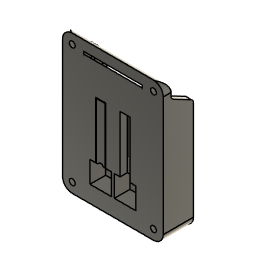
makita_10.8v_v38 v10 (Autodesk Fusion 360 design; units mm, degrees)
Autodesk Fusion 360 part; units mm, degrees
note: some values were not read from the file. Chosen so that the rebuilt part matches the saved one: a side; which face or edge a step refers to. Set by a fixed rule: which sketch regions a step uses.
(part 1 of 2)
sketch "スケッチ1" plane through (0, 0, 0) normal (0, 1, 0) x (1, 0, 0)
  line L0 (0, 0) -> (-15, 0)
  line L1 (-15, 0) -> (-15, 24)
  line L2 (-15, 24) -> (15, 24)
  line L3 (15, 24) -> (15, 0)
  line L4 (15, 0) -> (0, 0)
  line L5 (0, 0) -> (0, 36) construction
  line L6 (0, 0) -> (0, -57) construction
  line L7 (0.5, -4.15) -> (-0.5, -4.15)
  line L8 (-0.5, -4.15) -> (-0.5, -10.3)
  line L9 (-0.5, -10.3) -> (0.5, -10.3)
  line L10 (0.5, -10.3) -> (0.5, -4.15)
  line L11 (0.5, -4.15) -> (-0.5, -10.3) construction
  line L12 (-0.5, -4.15) -> (0.5, -10.3) construction
  line L13 (-6.75, 0) -> (-5.75, 0)
  line L14 (-5.75, 0) -> (-5.75, -19.4)
  line L15 (-5.75, -19.4) -> (-6.75, -19.4)
  line L16 (-6.75, -19.4) -> (-6.75, 0)
  line L17 (-6.75, -9.84) -> (-5.75, -9.84)
  line L18 (6.75, -19.4) -> (6.75, 0)
  line L19 (5.75, 0) -> (5.75, -19.4)
  line L20 (5.75, -19.4) -> (6.75, -19.4)
  line L21 (6.75, 0) -> (5.75, 0)
  line L22 (22.83, 24) -> (-22.83, 24)
  line L23 (-22.83, 24) -> (-22.83, -44.15)
  line L24 (-22.83, -44.15) -> (22.83, -44.15)
  line L25 (22.83, -44.15) -> (22.83, 24)
  line L26 (25.83, -44.15) -> (25.83, 27)
  line L27 (25.83, 27) -> (-25.83, 27)
  line L28 (-25.83, 27) -> (-25.83, -44.15)
  line L29 (-22.83, -44.15) -> (-25.83, -44.15)
  line L30 (22.83, -44.15) -> (25.83, -44.15)
  line L31 (-22.83, 1) -> (-18.63, 1)
  line L32 (-18.63, 1) -> (-18.63, -25)
  line L33 (-18.63, -25) -> (-22.83, -25)
  line L34 (-18.63, 1) -> (-18.63, 24)
  line L35 (18.63, 1) -> (18.63, 24)
  line L36 (22.83, 1) -> (18.63, 1)
  line L37 (18.63, 1) -> (18.63, -25)
  line L38 (18.63, -25) -> (22.83, -25)
  line L39 (6.75, -9.84) -> (5.75, -9.84)
  point P0 (0, -7.225)
  point P1 (0, 1.51)
  dimension "d1" = 30
  dimension "d2" = 24
  dimension "d3" = 1
  dimension "d4" = 1
  dimension "d5" = 6.15
  dimension "d6" = 19.4
  dimension "d7" = 4.15
  dimension "d8" = 5.25
  dimension "d9" = 9.56
  dimension "d10" = 45.66
  dimension "d11" = 44.15
  dimension "d12" = 3
  dimension "d13" = 1
  dimension "d14" = 26
  dimension "d15" = 7.2
  constraint coincident L0.start L4.end
  constraint horizontal L0
  constraint perpendicular L0 L1
  constraint perpendicular L1 L2
  constraint perpendicular L2 L3
  constraint perpendicular L1 L4
  constraint perpendicular L2 L5
  constraint perpendicular L0 L6
  constraint perpendicular L7 L8
  constraint parallel L7 L9
  constraint parallel L8 L10
  constraint horizontal L7
  constraint coincident L11 P0
  constraint coincident L12 P0
  constraint coincident L6 P0
  constraint horizontal L13
  constraint vertical L14
  constraint horizontal L15
  constraint vertical L16
  constraint coincident L0 L13.start
  constraint coincident L16 L17.start
  constraint coincident L14 L17.end
  constraint perpendicular L16 L17
  constraint symmetric L6 L13.start L18.end
  constraint symmetric L6 L13.end L19.start
  constraint symmetric L6 L14.end L19.end
  constraint symmetric L6 L15.end L18.start
  constraint perpendicular L22 L23
  constraint parallel L22 L24
  constraint parallel L23 L25
  constraint horizontal L22
  constraint coincident L6 P1
  constraint symmetric L6 L23 L25
  constraint collinear L2 L22
  constraint coincident L23 L31.start
  constraint perpendicular L23 L31
  constraint perpendicular L31 L32
  constraint coincident L23 L33.end
  constraint perpendicular L23 L33
  constraint coincident L22 L34.end
  constraint perpendicular L22 L34
  constraint symmetric L5 L31.start L36.start
  constraint symmetric L5 L31.end L35.start
  constraint symmetric L5 L32.end L37.end
  constraint symmetric L5 L33.end L38.end
  constraint symmetric L5 L34.end L35.end
  constraint vertical L6
  constraint symmetric L6 L17.start L39.start
  constraint symmetric L6 L17.end L39.end
  measures "d1" distance of L1 L3
  measures "d2" vertical distance of L0.end L1.end
  measures "d3" horizontal distance of L8.end L9.end
  measures "d4" horizontal distance of L14.end L15.end
  measures "d5" vertical distance of L7.end L8.end
  measures "d6" vertical distance of L13.start L15.end
  measures "d7" distance of L4 L7
  measures "d8" distance of L8 L14
  measures "d9" distance of L15 L17
  measures "d10" horizontal distance of L23.end L24.end
  measures "d11" distance of L4 L24
  measures "d13" distance of L0 L31
  measures "d14" vertical distance of L31.end L32.end
  measures "d15" distance of L28 L32
extrude "押し出し1" add sketch "スケッチ1" along normal blind 8 contours L0 L1 L2 L3 L4 L13 L21 L22 makes body 1
extrude "押し出し2" add sketch "スケッチ1" along normal blind 11.5 contours L2 L22 L23 L25 L26 L27 L28 L29 L30 | L23 L31 L32 L33 | L25 L36 L37 L38 bodies 1
extrude "押し出し3" cut sketch "スケッチ1" along normal blind 6.5 contours L22 L23 L31 L34 | L22 L25 L35 L36 | L23 L31 L32 L33 | L25 L36 L37 L38 bodies 1
extrude "押し出し4" add sketch "スケッチ1" against normal blind 4 contours L0 L1 L3 L4 L14 L15 L16 L18 L19 L20 L22 L23 L24 L25 L32 L33 L34 L35 L37 L38 | L0 L1 L2 L3 L4 L13 L21 L22 | L0 L13 L14 L16 L17 | L4 L18 L19 L21 L39 | L14 L15 L16 L17 | L18 L19 L20 L39 | L2 L22 L23 L25 L26 L27 L28 L29 L30 | L22 L23 L31 L34 | L22 L25 L35 L36 | L23 L31 L32 L33 | L25 L36 L37 L38 | L7 L8 L9 L10 bodies 1
extrude "押し出し5" cut sketch "スケッチ1" against normal up to surface (4 mm away) contours L14 L15 L16 L17 | L18 L19 L20 L39 bodies 1
sketch "スケッチ2" plane through (0, 0, 0) normal (0, 1, 0) x (-1, 0, 0)
  line L0 (-5.75, 19.4) -> (-5.75, 9.84)
  line L1 (-5.75, 9.84) -> (-6.75, 9.84)
  line L2 (-6.75, 9.84) -> (-6.75, 19.4)
  line L3 (-6.75, 19.4) -> (-5.75, 19.4)
  line L4 (5.75, 19.4) -> (6.75, 19.4)
  line L5 (6.75, 19.4) -> (6.75, 9.84)
  line L6 (6.75, 9.84) -> (5.75, 9.84)
  line L7 (5.75, 9.84) -> (5.75, 19.4)
  line L8 (-22.83, 44.15) -> (-22.83, -24)
  line L9 (-22.83, -24) -> (-15, -24)
  line L10 (-15, -24) -> (-15, 0)
  line L11 (-15, 0) -> (0, 0)
  line L12 (0, 0) -> (5.75, 0)
  line L13 (5.75, 0) -> (6.75, 0)
  line L14 (6.75, 0) -> (15, 0)
  line L15 (15, 0) -> (15, -24)
  line L16 (15, -24) -> (22.83, -24)
  line L17 (22.83, -24) -> (22.83, 44.15)
  line L18 (22.83, 44.15) -> (-22.83, 44.15)
  line L19 (6.75, 19.4) -> (6.75, 9.84)
  line L20 (5.75, 9.84) -> (5.75, 19.4)
  line L21 (-5.75, 19.4) -> (-5.75, 9.84)
  line L22 (-6.75, 9.84) -> (-6.75, 19.4)
  line L23 (8.175, 21.4) -> (4.325, 21.4)
  line L24 (4.325, 21.4) -> (4.325, 0)
  line L25 (4.325, 0) -> (8.175, 0)
  line L26 (8.175, 0) -> (8.175, 21.4)
  line L27 (6.25, 9.84) -> (6.25, 19.4) construction
  line L28 (0, 0) -> (0, 25.4511) construction
  line L29 (-8.175, 0) -> (-8.175, 21.4)
  line L30 (-4.325, 21.4) -> (-4.325, 0)
  line L31 (-8.175, 21.4) -> (-4.325, 21.4)
  dimension "d26" = 3.85
  dimension "d27" = 2
  constraint horizontal L23
  constraint vertical L24
  constraint horizontal L25
  constraint vertical L26
  constraint coincident L12 L24.end
  constraint midpoint L6 L27.start
  constraint midpoint L4 L27.end
  constraint symmetric L24 L26 L27
  constraint coincident L11.end L12.start
  constraint perpendicular L11 L28
  constraint symmetric L23.start L28 L29.end
  constraint symmetric L23.end L28 L30.start
  constraint symmetric L24.end L28 L30.end
  constraint symmetric L25.end L28 L29.start
  measures "d26" horizontal distance of L23.start L23.end
  measures "d27" distance of L4 L23
extrude "押し出し6" add sketch "スケッチ2" along normal blind 2 contours L11 L29 L30 L31 | L12 L13 L14 L23 L24 L25 L26 bodies 1
chamfer "面取り1" distance 1.5 angle 45 2 edges at (-6.25, 2, 21.4) (6.25, 2, 21.4) on bodies 1
chamfer "面取り2" distance 1 angle 45 4 edges at (-4.325, 1.25, 20.65) (-8.175, 1.25, 20.65) (4.325, 1.25, 20.65) (8.175, 1.25, 20.65) on bodies 1
ref_plane "作業平面1" through (0, 3.75, 8.575) normal (1, 0, 0) x (0, 0, -1)
sketch "スケッチ3" plane through (0, 4.75, 8.575) normal (1, 0, 0) x (0, 0, -1)
  line L0 (-35.575, -4.75) -> (-35.575, 4.5) construction
  line L1 (-35.575, -4.75) -> (8.575, -4.75)
  line L2 (-30.425, -4.75) -> (-30.425, -9.25)
  line L3 (-30.425, -9.25) -> (-19.425, -4.75)
  point P0 (-35.575, -4.75)
  point P1 (8.575, 3.25)
  point P2 (8.575, -4.75)
  dimension "d33" = 4.5
  dimension "d34" = 11
  dimension "d45" = 28
  constraint coincident P0 L0.start
  constraint vertical L0
  constraint coincident P2 L1.end
  constraint coincident L1 L2.start
  constraint perpendicular L1 L2
  constraint coincident L1 L3.end
  measures "d33" vertical distance of L2.start L2.end
  measures "d34" horizontal distance of L2.start L3.end
  measures "d45" horizontal distance of P2 L3.end
extrude "押し出し7" cut sketch "スケッチ3" along normal mid plane 30 bodies 1
fillet "フィレット1" radius 2 2 edges at (20.73, 6.5, 25) (-20.73, 6.5, 25) on bodies 1
fillet "フィレット2" radius 5 4 edges at (-25.83, 3.75, -27) (25.83, 3.75, -27) (-22.83, 5.75, -24) (22.83, 5.75, -24) on bodies 1
sketch "スケッチ4" plane through (0, -4, 0) normal (0, -1, 0) x (1, 0, 0)
  line L0 (6.75, 19.4) -> (6.75, 9.84)
  line L1 (6.75, 9.84) -> (5.75, 9.84)
  line L2 (5.75, 9.84) -> (5.75, 19.4)
  line L3 (5.75, 19.4) -> (6.75, 19.4)
  line L4 (-5.75, 9.84) -> (-6.75, 9.84)
  line L5 (-6.75, 9.84) -> (-6.75, 19.4)
  line L6 (-6.75, 19.4) -> (-5.75, 19.4)
  line L7 (-5.75, 19.4) -> (-5.75, 9.84)
  arc A0 (20.83, -27) -> (25.83, -22) centre (20.83, -22) ccw
  line L8 (25.83, -22) -> (25.83, 44.15)
  line L9 (25.83, 44.15) -> (-25.83, 44.15)
  line L10 (-25.83, 44.15) -> (-25.83, -22)
  arc A1 (-25.83, -22) -> (-20.83, -27) centre (-20.83, -22) ccw
  line L11 (-20.83, -27) -> (20.83, -27)
  line L12 (-5.75, 19.4) -> (-5.75, 9.84)
  line L13 (-6.75, 9.84) -> (-6.75, 19.4)
  line L14 (-6.75, 19.4) -> (-5.75, 19.4)
  line L15 (-5.75, 9.84) -> (-6.75, 9.84)
  line L16 (5.75, 9.84) -> (5.75, 19.4)
  line L17 (6.75, 19.4) -> (6.75, 9.84)
  line L18 (5.75, 19.4) -> (6.75, 19.4)
  line L19 (6.75, 9.84) -> (5.75, 9.84)
  line L20 (-5.5, 9.59) -> (-7, 9.59)
  line L21 (-7, 9.59) -> (-7, 19.65)
  line L22 (-7, 19.65) -> (-5.5, 19.65)
  line L23 (-5.5, 19.65) -> (-5.5, 9.59)
  line L24 (7, 9.59) -> (5.5, 9.59)
  line L25 (5.5, 9.59) -> (5.5, 19.65)
  line L26 (5.5, 19.65) -> (7, 19.65)
  line L27 (7, 19.65) -> (7, 9.59)
  line L28 (-15, 37.7778) -> (-15, 39)
  line L29 (-15, 39) -> (15, 39)
  line L30 (15, 39) -> (15, 37.7778)
  line L31 (15, 37.7778) -> (-15, 37.7778)
  dimension "d40" = 0.25
  dimension "d41" = 0.25
extrude "押し出し8" cut sketch "スケッチ4" against normal up to surface (6 mm away) contours L20 L21 L22 L23 | L24 L25 L26 L27 bodies 1
sketch "スケッチ5" plane through (25.83, 0, 0) normal (1, 0, 0) x (0, 0, -1)
  line L0 (22, -4) -> (22, 11.5)
  line L1 (22, 11.5) -> (-44.15, 11.5)
  line L2 (-44.15, 11.5) -> (-44.15, -4)
  line L3 (-44.15, -4) -> (22, -4)
  line L4 (19, 11.5) -> (19, 0)
  line L5 (19, 0) -> (-44.15, 0)
  line L6 (-44.15, 0) -> (-44.15, 11.5)
  line L7 (-44.15, 11.5) -> (-25, 11.5)
  line L8 (-25, 11.5) -> (-25, 8.5)
  arc A0 (-25, 8.5) -> (-23, 6.5) centre (-23, 8.5) ccw
  line L9 (-23, 6.5) -> (1, 6.5)
  line L10 (1, 6.5) -> (1, 11.5)
  line L11 (1, 11.5) -> (19, 11.5)
  line L12 (-36.15, 0) -> (-30.15, 11.5)
  dimension "d46" = 8
  dimension "d47" = 14
  constraint coincident L5 L12.start
  constraint coincident L7 L12.end
  measures "d46" horizontal distance of L5.end L12.start
  measures "d47" horizontal distance of L1.end L12.end
extrude "押し出し9" cut sketch "スケッチ5" against normal up to surface (51.66 mm away) contours L1 L2 L5 L6 L7 L12 bodies 1
fillet "フィレット3" radius 2 4 edges at (-24.33, 11.5, 30.15) (24.33, 11.5, 30.15) (24.33, 0, 36.15) (-24.33, 0, 36.15) on bodies 1
fillet "フィレット4" radius 5 3 edges at (-25.83, -2, 44.15) (25.83, -2, 44.15) (0, 0, 44.15) on bodies 1
extrude "押し出し10" add sketch "スケッチ1" along normal blind 7 separate body contours L14 L15 L16 L17 | L18 L19 L20 L39 makes body 2 at (6.75, 2.3333, 16.2133) makes body 3 at (-5.75, 2.3333, 13.0267)
extrude "押し出し11" add sketch "スケッチ1" against normal up to surface (4 mm away) contours L14 L15 L16 L17 | L18 L19 L20 L39 bodies 2 3
sketch "スケッチ6" plane through (0, -4, 0) normal (0, -1, 0) x (1, 0, 0)
  line L0 (-15, 37.7778) -> (-15, 39)
  line L1 (-15, 39) -> (15, 39)
  line L2 (15, 39) -> (15, 37.7778)
  line L3 (15, 37.7778) -> (-15, 37.7778)
  line L4 (7, 19.65) -> (7, 9.59)
  line L5 (7, 9.59) -> (5.5, 9.59)
  line L6 (5.5, 9.59) -> (5.5, 19.65)
  line L7 (5.5, 19.65) -> (7, 19.65)
  line L8 (-5.5, 19.65) -> (-5.5, 9.59)
  line L9 (-5.5, 9.59) -> (-7, 9.59)
  line L10 (-7, 9.59) -> (-7, 19.65)
  line L11 (-7, 19.65) -> (-5.5, 19.65)
  arc A0 (25.83, 39.15) -> (20.83, 44.15) centre (20.83, 39.15) ccw
  arc A1 (-20.83, 44.15) -> (-25.83, 39.15) centre (-20.83, 39.15) ccw
  line L12 (-25.83, 39.15) -> (-25.83, -22)
  arc A2 (-25.83, -22) -> (-20.83, -27) centre (-20.83, -22) ccw
  line L13 (-20.83, -27) -> (20.83, -27)
  arc A3 (20.83, -27) -> (25.83, -22) centre (20.83, -22) ccw
  line L14 (25.83, -22) -> (25.83, 39.15)
  line L15 (-6.75, 0) -> (-5.75, 0)
  line L16 (-5.75, 0) -> (0, 0)
  line L17 (0, 0) -> (15, 0)
  line L18 (15, 0) -> (15, -24)
  line L19 (15, -24) -> (-15, -24)
  line L20 (-15, -24) -> (-15, 0)
  line L21 (-15, 0) -> (-6.75, 0)
  line L22 (5.5, 9.59) -> (5.5, -20.6633)
  line L23 (5.5, -20.6633) -> (7, -20.6633)
  line L24 (7, -20.6633) -> (7, 9.59)
  line L25 (0, 0) -> (0, -24)
  line L26 (-5.5, 9.59) -> (-5.5, -20.6633)
  line L27 (-7, -20.6633) -> (-7, 9.59)
  line L28 (-5.5, -20.6633) -> (-7, -20.6633)
  line L29 (20.83, 44.15) -> (-20.83, 44.15)
  constraint coincident L5.end L6.start
  constraint perpendicular L5 L22
  constraint perpendicular L4 L23
  constraint coincident L4.end L5.start
  constraint perpendicular L5 L24
  constraint coincident L16.end L17.start
  constraint midpoint L19 L25.end
  constraint symmetric L5.end L25 L8.end
  constraint symmetric L22.end L25 L26.end
  constraint symmetric L23.end L25 L27.start
  constraint symmetric L4.end L25 L9.end
extrude "押し出し12" cut sketch "スケッチ6" against normal up to surface (11 mm away) contours L5 L17 L22 L24 | L17 L22 L23 L24 | L15 L16 L21 L26 L27 L28 | L9 L15 L16 L21 L26 L27 bodies 1
extrude "押し出し13" add 2 faces at (6.4167, -0.3333, 9.84) (-6.0833, 3.3333, 9.84) along direction (0, 0, -1) up to surface end surface through (-5.5, -4, -20.6633) normal (0, 0, 1) offset -0.25 on bodies 2 3 bodies 2 3
chamfer "面取り3" distance 1 angle 45 2 edges at (-6.25, 7, 19.4) (6.25, 7, 19.4) on bodies 2 3
sketch "スケッチ7" plane through (0, -4, 0) normal (0, -1, 0) x (1, 0, 0)
  line L0 (-7, -20.6633) -> (-7, 9.59)
  line L1 (-7, 9.59) -> (-7, 19.65)
  line L2 (-7, 19.65) -> (-5.5, 19.65)
  line L3 (-5.5, 19.65) -> (-5.5, 9.59)
  line L4 (-5.5, 9.59) -> (-5.5, -20.6633)
  line L5 (-5.5, -20.6633) -> (-7, -20.6633)
  line L6 (5.5, -20.6633) -> (5.5, 19.65)
  line L7 (5.5, 19.65) -> (7, 19.65)
  line L8 (7, 19.65) -> (7, -20.6633)
  line L9 (7, -20.6633) -> (5.5, -20.6633)
  line L10 (-15, 37.7778) -> (-15, 39)
  line L11 (-15, 39) -> (15, 39)
  line L12 (15, 39) -> (15, 37.7778)
  line L13 (15, 37.7778) -> (-15, 37.7778)
  arc A0 (25.83, 39.15) -> (20.83, 44.15) centre (20.83, 39.15) ccw
  arc A1 (-20.83, 44.15) -> (-25.83, 39.15) centre (-20.83, 39.15) ccw
  line L14 (-25.83, 39.15) -> (-25.83, -22)
  arc A2 (-25.83, -22) -> (-20.83, -27) centre (-20.83, -22) ccw
  line L15 (-20.83, -27) -> (20.83, -27)
  arc A3 (20.83, -27) -> (25.83, -22) centre (20.83, -22) ccw
  line L16 (25.83, -22) -> (25.83, 39.15)
  line L17 (-6.75, 0) -> (-5.75, 0)
  line L18 (-5.75, 0) -> (0, 0)
  line L19 (0, 0) -> (15, 0)
  line L20 (15, 0) -> (15, -24)
  line L21 (15, -24) -> (-15, -24)
  line L22 (-15, -24) -> (-15, 0)
  line L23 (-15, 0) -> (-6.75, 0)
  line L24 (5.75, 19.4) -> (5.75, -20.4133)
  line L25 (5.75, -20.4133) -> (6.75, -20.4133)
  line L26 (6.75, -20.4133) -> (6.75, 19.4)
  line L27 (6.75, 19.4) -> (5.75, 19.4)
  line L28 (-5.75, 19.4) -> (-6.75, 19.4)
  line L29 (-6.75, 19.4) -> (-6.75, -20.4133)
  line L30 (-6.75, -20.4133) -> (-5.75, -20.4133)
  line L31 (-5.75, -20.4133) -> (-5.75, 19.4)
  line L32 (0, 0) -> (0, -24)
  line L33 (-15, -14.4133) -> (15, -14.4133) construction
  line L34 (-6.25, -20.4133) -> (-6.25, 0) construction
  line L35 (-0.75, -10.4133) -> (-11.75, -10.4133)
  line L36 (-11.75, -10.4133) -> (-11.75, -18.4133)
  line L37 (-11.75, -18.4133) -> (-0.75, -18.4133)
  line L38 (-0.75, -18.4133) -> (-0.75, -10.4133)
  line L39 (-0.75, -10.4133) -> (-11.75, -18.4133) construction
  line L40 (-11.75, -10.4133) -> (-0.75, -18.4133) construction
  line L41 (0.75, -10.4133) -> (11.75, -10.4133)
  line L42 (11.75, -10.4133) -> (11.75, -18.4133)
  line L43 (0.75, -18.4133) -> (0.75, -10.4133)
  line L44 (11.75, -18.4133) -> (0.75, -18.4133)
  line L45 (20.83, 44.15) -> (-20.83, 44.15)
  point P0 (-6.25, -14.4133)
  dimension "d63" = 6
  dimension "d64" = 11
  dimension "d65" = 8
  constraint coincident L18.end L19.start
  constraint midpoint L21 L32.end
  constraint coincident L22 L33.start
  constraint coincident L20 L33.end
  constraint perpendicular L20 L33
  constraint midpoint L30 L34.start
  constraint midpoint L17 L34.end
  constraint perpendicular L35 L36
  constraint parallel L35 L37
  constraint parallel L36 L38
  constraint horizontal L35
  constraint coincident L39 P0
  constraint coincident L40 P0
  constraint coincident L33 P0
  constraint coincident L34 P0
  constraint symmetric L32 L35.start L41.start
  constraint symmetric L32 L35.end L41.end
  constraint symmetric L32 L36.end L42.end
  constraint symmetric L32 L37.end L43.start
  measures "d63" distance of L30 L33
  measures "d64" distance of L36.end L37.end
  measures "d65" distance of L35.end L36.end
extrude "押し出し15" cut sketch "スケッチ7" against normal up to surface (11 mm away) contours L0 L35 L36 L37 | L4 L35 L37 L38 | L6 L41 L43 L44 | L8 L41 L42 L44 bodies 1
sketch "スケッチ8" plane through (-6.75, 0, 0) normal (-1, 0, 0) x (0, 0, 1)
  line L0 (19.4, 6) -> (18.4, 7)
  line L1 (18.4, 7) -> (-20.4133, 7)
  line L2 (-20.4133, 7) -> (-20.4133, -4)
  line L3 (-20.4133, -4) -> (19.4, -4)
  line L4 (19.4, -4) -> (19.4, 6)
  line L5 (-18.4133, -4) -> (-10.4133, -4)
  line L6 (-18.4133, -4) -> (-10.4133, -4)
  line L7 (-10.4133, -4) -> (-10.4133, 7)
  line L8 (-10.4133, 7) -> (-18.4133, 7)
  line L9 (-18.4133, 7) -> (-18.4133, -4)
  line L10 (-18.4133, 7) -> (-10.4133, -4) construction
  line L11 (-10.4133, 7) -> (-18.4133, -4) construction
  circle A0 centre (-14.4133, 1.5) radius 1.6
  dimension "d68" = 3.2
  constraint coincident L8.end L9.start
  constraint coincident L5.end L6.end
  constraint coincident L7.end L8.start
  constraint coincident L5.start L6.start
  constraint midpoint L11 A0.centre
  measures "d68" diameter of A0
extrude "押し出し16" cut sketch "スケッチ8" against normal through all contours A0 bodies 2 3
ref_plane "作業平面2" through (0, -4.2, 8.575) normal (0, -1, 0) x (0, 0, -1)
sketch "スケッチ9" plane through (0, -4.2, 8.575) normal (0, -1, 0) x (1, 0, 0)
  arc A0 (25.83, 30.575) -> (20.83, 35.575) centre (20.83, 30.575) ccw
  line L0 (25.83, -30.575) -> (25.83, 30.575)
  line L1 (-20.83, -35.575) -> (20.83, -35.575)
  arc A1 (20.83, -35.575) -> (25.83, -30.575) centre (20.83, -30.575) ccw
  arc A2 (-25.83, -30.575) -> (-20.83, -35.575) centre (-20.83, -30.575) ccw
  line L2 (-25.83, 30.575) -> (-25.83, -30.575)
  arc A3 (-20.83, 35.575) -> (-25.83, 30.575) centre (-20.83, 30.575) ccw
  line L3 (11.75, -18.9883) -> (11.75, -26.9883)
  line L4 (0.75, -26.9883) -> (0.75, -18.9883)
  line L5 (-0.75, -18.9883) -> (-0.75, -26.9883)
  line L6 (-11.75, -26.9883) -> (-11.75, -18.9883)
  line L7 (11.75, -18.9883) -> (0.75, -18.9883)
  line L8 (0.75, -26.9883) -> (11.75, -26.9883)
  line L9 (-0.75, -18.9883) -> (-11.75, -18.9883)
  line L10 (-11.75, -26.9883) -> (-0.75, -26.9883)
  line L11 (20.83, 35.575) -> (-20.83, 35.575)
  constraint coincident L3.start L7.start
  constraint coincident L4.end L7.end
  constraint coincident L4.start L8.start
  constraint coincident L3.end L8.end
  constraint coincident L5.start L9.start
  constraint coincident L6.end L9.end
  constraint coincident L6.start L10.start
  constraint coincident L5.end L10.end
extrude "押し出し17" add sketch "スケッチ9" along normal blind 3 separate body makes body 4
sketch "スケッチ10" plane through (0, -4, 0) normal (0, -1, 0) x (1, 0, 0)
  line L0 (-7, -18.4133) -> (-11.75, -18.4133)
  line L1 (-11.75, -18.4133) -> (-11.75, -10.4133)
  line L2 (-11.75, -10.4133) -> (-7, -10.4133)
  line L3 (-7, -10.4133) -> (-7, 9.59)
  line L4 (-7, 9.59) -> (-7, 19.65)
  line L5 (-7, 19.65) -> (-5.5, 19.65)
  line L6 (-5.5, 19.65) -> (-5.5, 9.59)
  line L7 (-5.5, 9.59) -> (-5.5, -10.4133)
  line L8 (-5.5, -10.4133) -> (-0.75, -10.4133)
  line L9 (-0.75, -10.4133) -> (-0.75, -18.4133)
  line L10 (-0.75, -18.4133) -> (-5.5, -18.4133)
  line L11 (-5.5, -18.4133) -> (-5.5, -20.6633)
  line L12 (-5.5, -20.6633) -> (-7, -20.6633)
  line L13 (-7, -20.6633) -> (-7, -18.4133)
  line L14 (5.5, -18.4133) -> (0.75, -18.4133)
  line L15 (0.75, -18.4133) -> (0.75, -10.4133)
  line L16 (0.75, -10.4133) -> (5.5, -10.4133)
  line L17 (5.5, -10.4133) -> (5.5, 19.65)
  line L18 (5.5, 19.65) -> (7, 19.65)
  line L19 (7, 19.65) -> (7, -10.4133)
  line L20 (7, -10.4133) -> (11.75, -10.4133)
  line L21 (11.75, -10.4133) -> (11.75, -18.4133)
  line L22 (11.75, -18.4133) -> (7, -18.4133)
  line L23 (7, -18.4133) -> (7, -20.6633)
  line L24 (7, -20.6633) -> (5.5, -20.6633)
  line L25 (5.5, -20.6633) -> (5.5, -18.4133)
  line L26 (-15, 37.7778) -> (-15, 39)
  line L27 (-15, 39) -> (15, 39)
  line L28 (15, 39) -> (15, 37.7778)
  line L29 (15, 37.7778) -> (-15, 37.7778)
  arc A0 (25.83, 39.15) -> (20.83, 44.15) centre (20.83, 39.15) ccw
  arc A1 (-20.83, 44.15) -> (-25.83, 39.15) centre (-20.83, 39.15) ccw
  line L30 (-25.83, 39.15) -> (-25.83, -22)
  arc A2 (-25.83, -22) -> (-20.83, -27) centre (-20.83, -22) ccw
  line L31 (-20.83, -27) -> (20.83, -27)
  arc A3 (20.83, -27) -> (25.83, -22) centre (20.83, -22) ccw
  line L32 (25.83, -22) -> (25.83, 39.15)
  arc A4 (25.83, 39.15) -> (20.83, 44.15) centre (20.83, 39.15) ccw
  arc A5 (-20.83, 44.15) -> (-25.83, 39.15) centre (-20.83, 39.15) ccw
  arc A6 (-25.83, -22) -> (-20.83, -27) centre (-20.83, -22) ccw
  arc A7 (20.83, -27) -> (25.83, -22) centre (20.83, -22) ccw
  circle A8 centre (-20.83, -22) radius 2.5
  circle A9 centre (20.83, -22) radius 2.5
  line L33 (20.83, 44.15) -> (-20.83, 44.15)
  circle A10 centre (-20.83, 39.15) radius 2.5
  circle A11 centre (20.83, 39.15) radius 2.5
  dimension "d73" = 5
  constraint concentric A2 A8
  constraint concentric A7 A9
  constraint equal A8 A9
  constraint concentric A5 A10
  constraint concentric A4 A11
  constraint equal A8 A10
  constraint equal A10 A11
  measures "d73" diameter of A8
extrude "押し出し18" cut sketch "スケッチ10" against normal blind 3 contours A8 | A9 | A10 | A11 bodies 1
sketch "スケッチ11" plane through (0, -4.2, 0) normal (0, 1, 0) x (-1, 0, 0)
  line L0 (-11.75, -18.4133) -> (-11.75, -10.4133)
  line L1 (-11.75, -10.4133) -> (-0.75, -10.4133)
  line L2 (-0.75, -10.4133) -> (-0.75, -18.4133)
  line L3 (-0.75, -18.4133) -> (-11.75, -18.4133)
  line L4 (0.75, -18.4133) -> (0.75, -10.4133)
  line L5 (0.75, -10.4133) -> (11.75, -10.4133)
  line L6 (11.75, -10.4133) -> (11.75, -18.4133)
  line L7 (11.75, -18.4133) -> (0.75, -18.4133)
  line L8 (20.83, 44.15) -> (-20.83, 44.15)
  arc A0 (-20.83, 44.15) -> (-25.83, 39.15) centre (-20.83, 39.15) ccw
  line L9 (-25.83, 39.15) -> (-25.83, -22)
  arc A1 (-25.83, -22) -> (-20.83, -27) centre (-20.83, -22) ccw
  line L10 (-20.83, -27) -> (20.83, -27)
  arc A2 (20.83, -27) -> (25.83, -22) centre (20.83, -22) ccw
  line L11 (25.83, -22) -> (25.83, 39.15)
  arc A3 (25.83, 39.15) -> (20.83, 44.15) centre (20.83, 39.15) ccw
  circle A4 centre (20.83, 39.15) radius 2.5
  circle A5 centre (-20.83, 39.15) radius 2.5
  circle A6 centre (20.83, -22) radius 2.5
  circle A7 centre (-20.83, -22) radius 2.5
  line L12 (20.83, -19.5) -> (19.0622, -20.2322)
  line L13 (19.0622, -20.2322) -> (18.33, -22)
  line L14 (18.33, -22) -> (19.0622, -23.7678)
  line L15 (19.0622, -23.7678) -> (20.83, -24.5)
  line L16 (20.83, -24.5) -> (22.5978, -23.7678)
  line L17 (22.5978, -23.7678) -> (23.33, -22)
  line L18 (23.33, -22) -> (22.5978, -20.2322)
  line L19 (22.5978, -20.2322) -> (20.83, -19.5)
  line L20 (-20.83, -19.5) -> (-22.5978, -20.2322)
  line L21 (-22.5978, -20.2322) -> (-23.33, -22)
  line L22 (-23.33, -22) -> (-22.5978, -23.7678)
  line L23 (-22.5978, -23.7678) -> (-20.83, -24.5)
  line L24 (-20.83, -24.5) -> (-19.0622, -23.7678)
  line L25 (-19.0622, -23.7678) -> (-18.33, -22)
  line L26 (-18.33, -22) -> (-19.0622, -20.2322)
  line L27 (-19.0622, -20.2322) -> (-20.83, -19.5)
  line L28 (20.83, 41.65) -> (19.0622, 40.9178)
  line L29 (19.0622, 40.9178) -> (18.33, 39.15)
  line L30 (18.33, 39.15) -> (19.0622, 37.3822)
  line L31 (19.0622, 37.3822) -> (20.83, 36.65)
  line L32 (20.83, 36.65) -> (22.5978, 37.3822)
  line L33 (22.5978, 37.3822) -> (23.33, 39.15)
  line L34 (23.33, 39.15) -> (22.5978, 40.9178)
  line L35 (22.5978, 40.9178) -> (20.83, 41.65)
  line L36 (-20.83, 41.65) -> (-22.5978, 40.9178)
  line L37 (-22.5978, 40.9178) -> (-23.33, 39.15)
  line L38 (-23.33, 39.15) -> (-22.5978, 37.3822)
  line L39 (-22.5978, 37.3822) -> (-20.83, 36.65)
  line L40 (-20.83, 36.65) -> (-19.0622, 37.3822)
  line L41 (-19.0622, 37.3822) -> (-18.33, 39.15)
  line L42 (-18.33, 39.15) -> (-19.0622, 40.9178)
  line L43 (-19.0622, 40.9178) -> (-20.83, 41.65)
  point P0 (20.83, -22)
  point P1 (-20.83, -22)
  point P2 (20.83, 39.15)
  point P3 (-20.83, 39.15)
  constraint coincident A6 L12.start
  constraint coincident P0 A2.centre
  constraint coincident P1 A1.centre
  constraint coincident A7 L20.start
  constraint coincident A4 L28.start
  constraint coincident P2 A3.centre
  constraint coincident P3 A0.centre
  constraint coincident A5 L36.start
extrude "押し出し19" add sketch "スケッチ11" along normal blind 2.7 contours L28 L29 L30 L31 L32 L33 L34 L35 | L36 L37 L38 L39 L40 L41 L42 L43 | L12 L13 L14 L15 L16 L17 L18 L19 | L20 L21 L22 L23 L24 L25 L26 L27 bodies 4
fillet "フィレット5" radius 0.5 32 edges at (-21.7139, -1.5, -24.1339) (-19.9461, -1.5, -24.1339) (-18.6961, -1.5, -22.8839) (-18.6961, -1.5, -21.1161) (-19.9461, -1.5, -19.8661) (-21.7139, -1.5, -19.8661) (-22.9639, -1.5, -21.1161) (-22.9639, -1.5, -22.8839) (19.9461, -1.5, -24.1339) (21.7139, -1.5, -24.1339) (22.9639, -1.5, -22.8839) (22.9639, -1.5, -21.1161) (21.7139, -1.5, -19.8661) (19.9461, -1.5, -19.8661) (18.6961, -1.5, -21.1161) (18.6961, -1.5, -22.8839) (-21.7139, -1.5, 37.0161) (-19.9461, -1.5, 37.0161) (-18.6961, -1.5, 38.2661) (-18.6961, -1.5, 40.0339) (-19.9461, -1.5, 41.2839) (-21.7139, -1.5, 41.2839) (-22.9639, -1.5, 40.0339) (-22.9639, -1.5, 38.2661) (19.9461, -1.5, 37.0161) (21.7139, -1.5, 37.0161) (22.9639, -1.5, 38.2661) (22.9639, -1.5, 40.0339) (21.7139, -1.5, 41.2839) (19.9461, -1.5, 41.2839) (18.6961, -1.5, 40.0339) (18.6961, -1.5, 38.2661) on bodies 4
sketch "Sketch12" plane through (0, -4, 0) normal (0, -1, 0) x (1, 0, 0)
  circle A0 centre (-20.83, -22) radius 2.5
  circle A1 centre (-20.83, 39.15) radius 2.5
  circle A2 centre (20.83, -22) radius 2.5
  circle A3 centre (20.83, 39.15) radius 2.5
  line L0 (-15, 37.7778) -> (-15, 39)
  line L1 (-15, 39) -> (15, 39)
  line L2 (15, 39) -> (15, 37.7778)
  line L3 (15, 37.7778) -> (-15, 37.7778)
  arc A4 (25.83, 39.15) -> (20.83, 44.15) centre (20.83, 39.15) ccw
  line L4 (20.83, 44.15) -> (-20.83, 44.15)
  arc A5 (-20.83, 44.15) -> (-25.83, 39.15) centre (-20.83, 39.15) ccw
  line L5 (-25.83, 39.15) -> (-25.83, -22)
  arc A6 (-25.83, -22) -> (-20.83, -27) centre (-20.83, -22) ccw
  line L6 (-20.83, -27) -> (20.83, -27)
  arc A7 (20.83, -27) -> (25.83, -22) centre (20.83, -22) ccw
  line L7 (25.83, -22) -> (25.83, 39.15)
  line L8 (7, -10.4133) -> (11.75, -10.4133)
  line L9 (11.75, -10.4133) -> (11.75, -18.4133)
  line L10 (11.75, -18.4133) -> (7, -18.4133)
  line L11 (7, -18.4133) -> (7, -20.6633)
  line L12 (7, -20.6633) -> (5.5, -20.6633)
  line L13 (5.5, -20.6633) -> (5.5, -18.4133)
  line L14 (5.5, -18.4133) -> (0.75, -18.4133)
  line L15 (0.75, -18.4133) -> (0.75, -10.4133)
  line L16 (0.75, -10.4133) -> (5.5, -10.4133)
  line L17 (5.5, -10.4133) -> (5.5, 19.65)
  line L18 (5.5, 19.65) -> (7, 19.65)
  line L19 (7, 19.65) -> (7, -10.4133)
  line L20 (-11.75, -10.4133) -> (-7, -10.4133)
  line L21 (-7, -10.4133) -> (-7, 9.59)
  line L22 (-7, 9.59) -> (-7, 19.65)
  line L23 (-7, 19.65) -> (-5.5, 19.65)
  line L24 (-5.5, 19.65) -> (-5.5, 9.59)
  line L25 (-5.5, 9.59) -> (-5.5, -10.4133)
  line L26 (-5.5, -10.4133) -> (-0.75, -10.4133)
  line L27 (-0.75, -10.4133) -> (-0.75, -18.4133)
  line L28 (-0.75, -18.4133) -> (-5.5, -18.4133)
  line L29 (-5.5, -18.4133) -> (-5.5, -20.6633)
  line L30 (-5.5, -20.6633) -> (-7, -20.6633)
  line L31 (-7, -20.6633) -> (-7, -18.4133)
  line L32 (-7, -18.4133) -> (-11.75, -18.4133)
  line L33 (-11.75, -18.4133) -> (-11.75, -10.4133)
  circle A8 centre (-20.83, 39.15) radius 1.5
  circle A9 centre (-20.83, -22) radius 1.5
  circle A10 centre (20.83, -22) radius 1.5
  circle A11 centre (20.83, 39.15) radius 1.5
  dimension "d84" = 3
  dimension "d85" = 3
  dimension "d86" = 3
  dimension "d87" = 3
  constraint concentric A1 A8
  constraint concentric A0 A9
  constraint concentric A2 A10
  constraint concentric A3 A11
  measures "d84" diameter of A8
  measures "d85" diameter of A9
  measures "d86" diameter of A10
  measures "d87" diameter of A11
extrude "Extrude20" add sketch "Sketch12" against normal up to surface (3 mm away) contours A0 | A1 | A2 | A3 bodies 1
chamfer "Chamfer4" distance 5 angle 45 4 edges at (-9.375, -4, -10.4133) (-3.125, -4, -10.4133) (3.125, -4, -10.4133) (9.375, -4, -10.4133) on bodies 1
sketch "Sketch13" plane through (0, -4, 0) normal (0, -1, 0) x (1, 0, 0)
  line L0 (-5.5, -5.4133) -> (-0.75, -5.4133)
  line L1 (-0.75, -5.4133) -> (-0.75, -18.4133)
  line L2 (-0.75, -18.4133) -> (-5.5, -18.4133)
  line L3 (-5.5, -18.4133) -> (-5.5, -20.6633)
  line L4 (-5.5, -20.6633) -> (-7, -20.6633)
  line L5 (-7, -20.6633) -> (-7, -18.4133)
  line L6 (-7, -18.4133) -> (-11.75, -18.4133)
  line L7 (-11.75, -18.4133) -> (-11.75, -5.4133)
  line L8 (-11.75, -5.4133) -> (-7, -5.4133)
  line L9 (-7, -5.4133) -> (-7, 9.59)
  line L10 (-7, 9.59) -> (-7, 19.65)
  line L11 (-7, 19.65) -> (-5.5, 19.65)
  line L12 (-5.5, 19.65) -> (-5.5, 9.59)
  line L13 (-5.5, 9.59) -> (-5.5, -5.4133)
  circle A0 centre (-20.83, -22) radius 1.5
  circle A1 centre (-20.83, 39.15) radius 1.5
  circle A2 centre (20.83, -22) radius 1.5
  circle A3 centre (20.83, 39.15) radius 1.5
  line L14 (-15, 37.7778) -> (-15, 39)
  line L15 (-15, 39) -> (15, 39)
  line L16 (15, 39) -> (15, 37.7778)
  line L17 (15, 37.7778) -> (-15, 37.7778)
  arc A4 (25.83, 39.15) -> (20.83, 44.15) centre (20.83, 39.15) ccw
  line L18 (20.83, 44.15) -> (-20.83, 44.15)
  arc A5 (-20.83, 44.15) -> (-25.83, 39.15) centre (-20.83, 39.15) ccw
  line L19 (-25.83, 39.15) -> (-25.83, -22)
  arc A6 (-25.83, -22) -> (-20.83, -27) centre (-20.83, -22) ccw
  line L20 (-20.83, -27) -> (20.83, -27)
  arc A7 (20.83, -27) -> (25.83, -22) centre (20.83, -22) ccw
  line L21 (25.83, -22) -> (25.83, 39.15)
  line L22 (7, -5.4133) -> (11.75, -5.4133)
  line L23 (11.75, -5.4133) -> (11.75, -18.4133)
  line L24 (11.75, -18.4133) -> (7, -18.4133)
  line L25 (7, -18.4133) -> (7, -20.6633)
  line L26 (7, -20.6633) -> (5.5, -20.6633)
  line L27 (5.5, -20.6633) -> (5.5, -18.4133)
  line L28 (5.5, -18.4133) -> (0.75, -18.4133)
  line L29 (0.75, -18.4133) -> (0.75, -5.4133)
  line L30 (0.75, -5.4133) -> (5.5, -5.4133)
  line L31 (5.5, -5.4133) -> (5.5, 19.65)
  line L32 (5.5, 19.65) -> (7, 19.65)
  line L33 (7, 19.65) -> (7, -5.4133)
  line L34 (-7, -10.4133) -> (-7, -5.4133) construction
  line L35 (-7, -5.4133) -> (-11.75, -5.4133) construction
  line L36 (-11.75, -5.4133) -> (-11.75, -10.4133) construction
  line L37 (-11.75, -10.4133) -> (-7, -10.4133) construction
  line L38 (-5.5, -5.4133) -> (-5.5, -10.4133) construction
  line L39 (-5.5, -10.4133) -> (-0.75, -10.4133) construction
  line L40 (-0.75, -10.4133) -> (-0.75, -5.4133) construction
  line L41 (-0.75, -5.4133) -> (-5.5, -5.4133) construction
  line L42 (5.5, -10.4133) -> (5.5, -5.4133) construction
  line L43 (5.5, -5.4133) -> (0.75, -5.4133) construction
  line L44 (0.75, -5.4133) -> (0.75, -10.4133) construction
  line L45 (0.75, -10.4133) -> (5.5, -10.4133) construction
  line L46 (7, -5.4133) -> (7, -10.4133) construction
  line L47 (7, -10.4133) -> (11.75, -10.4133) construction
  line L48 (11.75, -10.4133) -> (11.75, -5.4133) construction
  line L49 (11.75, -5.4133) -> (7, -5.4133) construction
  line L50 (-11.75, -5.4133) -> (11.75, -5.4133)
  line L51 (11.75, -5.4133) -> (11.75, -10.4133)
  line L52 (11.75, -10.4133) -> (-11.75, -10.4133)
  line L53 (-11.75, -10.4133) -> (-11.75, -5.4133)
  constraint horizontal L50
  constraint vertical L51
  constraint horizontal L52
  constraint vertical L53
  constraint coincident L47.end L48.start
  constraint coincident L7.end L8.start
extrude "Extrude21" cut sketch "Sketch13" against normal blind 11 contours L0 L1 L7 L8 L50 L52 L53 | L22 L23 L29 L30 L50 L51 L52 bodies 1
sketch "Sketch14" plane through (0, -4, 0) normal (0, -1, 0) x (1, 0, 0)
  line L0 (-5.5, -5.4133) -> (-0.75, -5.4133)
  line L1 (-0.75, -5.4133) -> (-0.75, -18.4133)
  line L2 (-0.75, -18.4133) -> (-5.5, -18.4133)
  line L3 (-5.5, -18.4133) -> (-5.5, -20.6633)
  line L4 (-5.5, -20.6633) -> (-7, -20.6633)
  line L5 (-7, -20.6633) -> (-7, -18.4133)
  line L6 (-7, -18.4133) -> (-11.75, -18.4133)
  line L7 (-11.75, -18.4133) -> (-11.75, -5.4133)
  line L8 (-11.75, -5.4133) -> (-7, -5.4133)
  line L9 (-7, -5.4133) -> (-7, 9.59)
  line L10 (-7, 9.59) -> (-7, 19.65)
  line L11 (-7, 19.65) -> (-5.5, 19.65)
  line L12 (-5.5, 19.65) -> (-5.5, 9.59)
  line L13 (-5.5, 9.59) -> (-5.5, -5.4133)
  circle A0 centre (-20.83, -22) radius 1.5
  circle A1 centre (-20.83, 39.15) radius 1.5
  circle A2 centre (20.83, -22) radius 1.5
  circle A3 centre (20.83, 39.15) radius 1.5
  line L14 (-15, 37.7778) -> (-15, 39)
  line L15 (-15, 39) -> (15, 39)
  line L16 (15, 39) -> (15, 37.7778)
  line L17 (15, 37.7778) -> (-15, 37.7778)
  arc A4 (25.83, 39.15) -> (20.83, 44.15) centre (20.83, 39.15) ccw
  line L18 (20.83, 44.15) -> (-20.83, 44.15)
  arc A5 (-20.83, 44.15) -> (-25.83, 39.15) centre (-20.83, 39.15) ccw
  line L19 (-25.83, 39.15) -> (-25.83, -22)
  arc A6 (-25.83, -22) -> (-20.83, -27) centre (-20.83, -22) ccw
  line L20 (-20.83, -27) -> (20.83, -27)
  arc A7 (20.83, -27) -> (25.83, -22) centre (20.83, -22) ccw
  line L21 (25.83, -22) -> (25.83, 39.15)
  line L22 (7, -5.4133) -> (11.75, -5.4133)
  line L23 (11.75, -5.4133) -> (11.75, -18.4133)
  line L24 (11.75, -18.4133) -> (7, -18.4133)
  line L25 (7, -18.4133) -> (7, -20.6633)
  line L26 (7, -20.6633) -> (5.5, -20.6633)
  line L27 (5.5, -20.6633) -> (5.5, -18.4133)
  line L28 (5.5, -18.4133) -> (0.75, -18.4133)
  line L29 (0.75, -18.4133) -> (0.75, -5.4133)
  line L30 (0.75, -5.4133) -> (5.5, -5.4133)
  line L31 (5.5, -5.4133) -> (5.5, 19.65)
  line L32 (5.5, 19.65) -> (7, 19.65)
  line L33 (7, 19.65) -> (7, -5.4133)
  line L34 (-7, 19.65) -> (-5.8, 19.65)
  line L35 (-5.8, 19.65) -> (-5.8, -10.35)
  line L36 (-5.8, -10.35) -> (-7, -10.35)
  line L37 (-7, -10.35) -> (-7, 19.65)
  dimension "d93" = 1.2
  dimension "d94" = 30
  constraint horizontal L34
  constraint vertical L35
  constraint horizontal L36
  constraint vertical L37
  constraint coincident L10.end L11.start
  measures "d93" distance of L10.end L34.end
  measures "d94" distance of L10.end L36.end
extrude "Extrude22" add sketch "Sketch14" along normal blind 7.3 separate body contours L9 L10 L11 L34 L35 L36 L37 makes body 5
move_body "Move1" bodies 5 to x (1, 0, 0) y (0, 1, 0) z (0, 0, 1) at (0, 11.09, 0)
sketch "Sketch16" plane through (0, 7, 0) normal (0, -1, 0) x (1, 0, 0)
  line L0 (7, -5.4133) -> (7, 0)
  line L1 (7, 0) -> (5.5, 0)
  line L2 (5.5, 0) -> (5.5, -5.4133)
  line L3 (5.5, -5.4133) -> (0.75, -5.4133)
  line L4 (0.75, -5.4133) -> (0.75, -18.4133)
  line L5 (0.75, -18.4133) -> (5.5, -18.4133)
  line L6 (5.5, -18.4133) -> (5.5, -20.6633)
  line L7 (5.5, -20.6633) -> (7, -20.6633)
  line L8 (7, -20.6633) -> (7, -18.4133)
  line L9 (7, -18.4133) -> (11.75, -18.4133)
  line L10 (11.75, -18.4133) -> (11.75, -10.4133)
  line L11 (11.75, -10.4133) -> (11.75, -5.4133)
  line L12 (11.75, -5.4133) -> (7, -5.4133)
  line L13 (7, -18.4133) -> (5.5, -18.4133)
  line L14 (-11.75, -5.4133) -> (-11.75, -18.4133)
  line L15 (-11.75, -18.4133) -> (-7, -18.4133)
  line L16 (-7, -18.4133) -> (-7, -20.6633)
  line L17 (-7, -20.6633) -> (-5.5, -20.6633)
  line L18 (-5.5, -20.6633) -> (-5.5, -18.4133)
  line L19 (-5.5, -18.4133) -> (-0.75, -18.4133)
  line L20 (-0.75, -18.4133) -> (-0.75, -5.4133)
  line L21 (-0.75, -5.4133) -> (-5.5, -5.4133)
  line L22 (-5.5, -5.4133) -> (-5.5, 0)
  line L23 (-5.5, 0) -> (-5.75, 0)
  line L24 (-5.75, 0) -> (-6.75, 0)
  line L25 (-6.75, 0) -> (-7, 0)
  line L26 (-7, 0) -> (-7, -5.4133)
  line L27 (-7, -5.4133) -> (-11.75, -5.4133)
  line L28 (-5.5, -18.4133) -> (-7, -18.4133)
  constraint coincident L8.end L9.start
  constraint coincident L5.end L6.start
  constraint coincident L18.end L19.start
  constraint coincident L15.end L16.start
extrude "Extrude23" add sketch "Sketch16" along normal blind 11 contours L6 L7 L8 L13 | L16 L17 L18 L28 bodies 1
sketch "Sketch17" plane through (0, -4, 0) normal (0, -1, 0) x (1, 0, 0)
  line L0 (-5.5, -5.4133) -> (-0.75, -5.4133)
  line L1 (-0.75, -5.4133) -> (-0.75, -18.4133)
  line L2 (-0.75, -18.4133) -> (-11.75, -18.4133)
  line L3 (-11.75, -18.4133) -> (-11.75, -5.4133)
  line L4 (-11.75, -5.4133) -> (-7, -5.4133)
  line L5 (-7, -5.4133) -> (-7, 9.59)
  line L6 (-7, 9.59) -> (-7, 19.65)
  line L7 (-7, 19.65) -> (-5.5, 19.65)
  line L8 (-5.5, 19.65) -> (-5.5, 9.59)
  line L9 (-5.5, 9.59) -> (-5.5, -5.4133)
  circle A0 centre (-20.83, -22) radius 1.5
  circle A1 centre (-20.83, 39.15) radius 1.5
  circle A2 centre (20.83, -22) radius 1.5
  circle A3 centre (20.83, 39.15) radius 1.5
  line L10 (-15, 37.7778) -> (-15, 39)
  line L11 (-15, 39) -> (15, 39)
  line L12 (15, 39) -> (15, 37.7778)
  line L13 (15, 37.7778) -> (-15, 37.7778)
  arc A4 (25.83, 39.15) -> (20.83, 44.15) centre (20.83, 39.15) ccw
  line L14 (20.83, 44.15) -> (-20.83, 44.15)
  arc A5 (-20.83, 44.15) -> (-25.83, 39.15) centre (-20.83, 39.15) ccw
  line L15 (-25.83, 39.15) -> (-25.83, -22)
  arc A6 (-25.83, -22) -> (-20.83, -27) centre (-20.83, -22) ccw
  line L16 (-20.83, -27) -> (20.83, -27)
  arc A7 (20.83, -27) -> (25.83, -22) centre (20.83, -22) ccw
  line L17 (25.83, -22) -> (25.83, 39.15)
  line L18 (7, -5.4133) -> (11.75, -5.4133)
  line L19 (11.75, -5.4133) -> (11.75, -18.4133)
  line L20 (11.75, -18.4133) -> (0.75, -18.4133)
  line L21 (0.75, -18.4133) -> (0.75, -5.4133)
  line L22 (0.75, -5.4133) -> (5.5, -5.4133)
  line L23 (5.5, -5.4133) -> (5.5, 19.65)
  line L24 (5.5, 19.65) -> (7, 19.65)
  line L25 (7, 19.65) -> (7, -5.4133)
  line L26 (-7, -5.4133) -> (-7, -7.4133) construction
  line L27 (-7, -7.4133) -> (-7.3638, -7.4133) construction
  line L28 (-7.3638, -7.4133) -> (-11.75, -7.4133) construction
  line L29 (-6.8, -5.4133) -> (-6.8, -7.4133)
  line L30 (-6.8, -7.4133) -> (-11.75, -7.4133)
  line L31 (-6.25, -18.4133) -> (-6.25, 19.65) construction
  line L32 (-6.8, -5.4133) -> (-6.8, 19.65)
  line L33 (-5.7, -7.4133) -> (-0.75, -7.4133)
  line L34 (-5.7, -5.4133) -> (-5.7, -7.4133)
  line L35 (-5.7, -5.4133) -> (-5.7, 19.65)
  line L36 (-11.75, -18.4133) -> (-0.75, -18.4133)
  line L37 (-0.75, -18.4133) -> (-0.75, -5.4133)
  line L38 (-0.75, -5.4133) -> (-5.5, -5.4133)
  line L39 (-5.5, -5.4133) -> (-5.5, 0)
  line L40 (-5.5, 0) -> (-5.75, 0)
  line L41 (-5.75, 0) -> (-6.75, 0)
  line L42 (-6.75, 0) -> (-7, 0)
  line L43 (-7, 0) -> (-7, -5.4133)
  line L44 (-7, -5.4133) -> (-11.75, -5.4133)
  line L45 (-11.75, -5.4133) -> (-11.75, -18.4133)
  line L46 (-5.7, 0) -> (-5.5, 0)
  line L47 (-6.8, 0) -> (-7, 0)
  line L48 (0, -27) -> (0, 44.15) construction
  line L49 (6.8, -5.4133) -> (6.8, 19.65)
  line L50 (6.8, -5.4133) -> (6.8, -7.4133)
  line L51 (6.8, -7.4133) -> (11.75, -7.4133)
  line L52 (5.7, -5.4133) -> (5.7, 19.65)
  line L53 (5.7, -7.4133) -> (0.75, -7.4133)
  line L54 (5.7, -5.4133) -> (5.7, -7.4133)
  line L55 (6.8, 0) -> (7, 0)
  line L56 (5.7, 0) -> (5.5, 0)
  line L57 (7, 0) -> (7, -5.4133)
  line L58 (7, -5.4133) -> (11.75, -5.4133)
  line L59 (11.75, -5.4133) -> (11.75, -18.4133)
  line L60 (11.75, -18.4133) -> (0.75, -18.4133)
  line L61 (0.75, -18.4133) -> (0.75, -5.4133)
  line L62 (0.75, -5.4133) -> (5.5, -5.4133)
  line L63 (5.5, -5.4133) -> (5.5, 0)
  line L64 (5.5, 0) -> (5.75, 0)
  line L65 (6.75, 0) -> (7, 0)
  line L66 (5.75, 0) -> (6.75, 0)
  dimension "d99" = 2
  dimension "d100" = -0.2
  constraint coincident L4.end L5.start
  constraint perpendicular L4 L26
  constraint perpendicular L26 L27
  constraint coincident L3 L28.end
  constraint perpendicular L3 L28
  constraint perpendicular L26 L30
  constraint midpoint L2 L31.start
  constraint midpoint L7 L31.end
  constraint coincident L7 L32.end
  constraint perpendicular L7 L32
  constraint symmetric L28.end L31 L33.end
  constraint symmetric L29.start L31 L34.start
  constraint symmetric L29.end L31 L33.start
  constraint symmetric L31 L32.end L35.end
  constraint coincident L40 L46.start
  constraint coincident L35 L46.start
  constraint coincident L39.end L40.start
  constraint coincident L32 L47.start
  constraint coincident L42 L47.start
  constraint coincident L42.end L43.start
  constraint midpoint L16 L48.start
  constraint midpoint L14 L48.end
  constraint symmetric L28.end L48 L51.end
  constraint symmetric L29.start L48 L49.start
  constraint symmetric L29.end L48 L50.end
  constraint symmetric L32.end L48 L49.end
  constraint symmetric L33.start L48 L53.start
  constraint symmetric L33.end L48 L53.end
  constraint symmetric L34.start L48 L52.start
  constraint symmetric L35.end L48 L52.end
  constraint symmetric L2.end L48 L19.end
  constraint symmetric L1.end L48 L20.end
  constraint symmetric L0.end L48 L21.end
  constraint symmetric L0.start L48 L22.end
  constraint symmetric L39.end L48 L56.end
  constraint symmetric L40.end L48 L64.end
  constraint symmetric L41.end L48 L65.start
  constraint symmetric L42.end L48 L55.end
  constraint symmetric L4.end L48 L18.start
  constraint symmetric L3.end L48 L18.end
  constraint symmetric L46.start L48 L56.start
  constraint symmetric L47.start L48 L55.start
  measures "d99" distance of L4.end L26.end
extrude "Extrude24" add sketch "Sketch17" against normal blind 11 contours L0 L1 L9 L33 L34 L35 L37 L38 L39 L40 L46 | L3 L4 L5 L29 L30 L32 L42 L43 L44 L45 L47 | L18 L19 L25 L49 L50 L51 L55 L57 L58 L59 L65 | L21 L22 L23 L52 L53 L54 L56 L61 L62 L63 L64 bodies 1
extrude "Extrude25" add sketch "Sketch17" against normal blind 6 contours L7 L8 L9 L35 L40 L46 | L5 L6 L7 L32 L42 L47 | L24 L25 L49 L55 L65 | L23 L24 L52 L56 L64 bodies 1
chamfer "Chamfer5" distance 1 angle 45 4 edges at (-6.8, 1.5, -7.4133) (-5.7, 1.5, -7.4133) (5.7, 1.5, -7.4133) (6.8, 1.5, -7.4133) on bodies 1
sketch "Sketch18" plane through (0, -4, 0) normal (0, -1, 0) x (1, 0, 0)
  line L0 (6.8, -6.4133) -> (7.8, -7.4133)
  line L1 (7.8, -7.4133) -> (11.75, -7.4133)
  line L2 (11.75, -7.4133) -> (11.75, -18.4133)
  line L3 (11.75, -18.4133) -> (0.75, -18.4133)
  line L4 (0.75, -18.4133) -> (0.75, -7.4133)
  line L5 (0.75, -7.4133) -> (4.7, -7.4133)
  line L6 (4.7, -7.4133) -> (5.7, -6.4133)
  line L7 (5.7, -6.4133) -> (5.7, 19.65)
  line L8 (5.7, 19.65) -> (6.8, 19.65)
  line L9 (6.8, 19.65) -> (6.8, -6.4133)
  arc A0 (25.83, 39.15) -> (20.83, 44.15) centre (20.83, 39.15) ccw
  line L10 (20.83, 44.15) -> (-20.83, 44.15)
  arc A1 (-20.83, 44.15) -> (-25.83, 39.15) centre (-20.83, 39.15) ccw
  line L11 (-25.83, 39.15) -> (-25.83, -22)
  arc A2 (-25.83, -22) -> (-20.83, -27) centre (-20.83, -22) ccw
  line L12 (-20.83, -27) -> (20.83, -27)
  arc A3 (20.83, -27) -> (25.83, -22) centre (20.83, -22) ccw
  line L13 (25.83, -22) -> (25.83, 39.15)
  line L14 (-15, 37.7778) -> (-15, 39)
  line L15 (-15, 39) -> (15, 39)
  line L16 (15, 39) -> (15, 37.7778)
  line L17 (15, 37.7778) -> (-15, 37.7778)
  circle A4 centre (20.83, 39.15) radius 1.5
  circle A5 centre (20.83, -22) radius 1.5
  circle A6 centre (-20.83, 39.15) radius 1.5
  circle A7 centre (-20.83, -22) radius 1.5
  line L18 (-5.7, -6.4133) -> (-4.7, -7.4133)
  line L19 (-4.7, -7.4133) -> (-0.75, -7.4133)
  line L20 (-0.75, -7.4133) -> (-0.75, -18.4133)
  line L21 (-0.75, -18.4133) -> (-11.75, -18.4133)
  line L22 (-11.75, -18.4133) -> (-11.75, -7.4133)
  line L23 (-11.75, -7.4133) -> (-7.8, -7.4133)
  line L24 (-7.8, -7.4133) -> (-6.8, -6.4133)
  line L25 (-6.8, -6.4133) -> (-6.8, 19.65)
  line L26 (-6.8, 19.65) -> (-5.7, 19.65)
  line L27 (-5.7, 19.65) -> (-5.7, -6.4133)
  line L28 (-1.15, -18.0133) -> (-11.35, -18.0133)
  line L29 (-11.35, -18.0133) -> (-11.35, -7.8133)
  line L30 (-11.35, -7.8133) -> (-7.6343, -7.8133)
  line L31 (-7.6343, -7.8133) -> (-6.4, -6.579)
  line L32 (-6.4, -6.579) -> (-6.4, 19.25)
  line L33 (-6.4, 19.25) -> (-6.1, 19.25)
  line L34 (-6.1, 19.25) -> (-6.1, -6.579)
  line L35 (-6.1, -6.579) -> (-4.8657, -7.8133)
  line L36 (-4.8657, -7.8133) -> (-1.15, -7.8133)
  line L37 (-1.15, -7.8133) -> (-1.15, -18.0133)
  line L38 (-6.4, -6.579) -> (-6.1, -6.579) construction
  line L39 (-6.25, -6.579) -> (-6.25, -7.8133) construction
  line L40 (-6.25, -7.8133) -> (-6.25, -9.8133) construction
  line L41 (-6.25, -9.8133) -> (-10.35, -9.8133)
  line L42 (-6.4, -6.579) -> (-6.1, -6.579)
  line L43 (-6.25, -9.8133) -> (-2.15, -9.8133)
  line L44 (-11.35, -7.8133) -> (-10.35, -7.8133) construction
  line L45 (-1.15, -7.8133) -> (-2.15, -7.8133) construction
  line L46 (-10.35, -9.8133) -> (-10.35, -15.7085)
  line L47 (-2.15, -9.8133) -> (-2.15, -15.7882)
  line L48 (-10.35, -15.7085) -> (-7.8571, -17.1099)
  line L49 (-4.5853, -17.1099) -> (-2.15, -15.7882)
  line L50 (-7.8571, -17.1099) -> (-4.5853, -17.1099)
  line L51 (0, -27) -> (0, 44.15) construction
  line L52 (6.1, -6.579) -> (4.8657, -7.8133)
  line L53 (4.8657, -7.8133) -> (1.15, -7.8133)
  line L54 (1.15, -7.8133) -> (1.15, -18.0133)
  line L55 (1.15, -18.0133) -> (11.35, -18.0133)
  line L56 (11.35, -18.0133) -> (11.35, -7.8133)
  line L57 (11.35, -7.8133) -> (7.6343, -7.8133)
  line L58 (7.6343, -7.8133) -> (6.4, -6.579)
  line L59 (4.5853, -17.1099) -> (2.15, -15.7882)
  line L60 (7.8571, -17.1099) -> (4.5853, -17.1099)
  line L61 (10.35, -15.7085) -> (7.8571, -17.1099)
  line L62 (10.35, -9.8133) -> (10.35, -15.7085)
  line L63 (6.25, -9.8133) -> (10.35, -9.8133)
  line L64 (6.25, -9.8133) -> (2.15, -9.8133)
  line L65 (2.15, -9.8133) -> (2.15, -15.7882)
  line L66 (6.4, -6.579) -> (6.1, -6.579) construction
  line L67 (6.4, -6.579) -> (6.1, -6.579)
  dimension "d106" = 0.4
  dimension "d107" = 2
  dimension "d108" = 1
  dimension "d109" = 1
  constraint midpoint L38 L39.start
  constraint perpendicular L38 L39
  constraint perpendicular L38 L40
  constraint perpendicular L29 L41
  constraint perpendicular L37 L43
  constraint perpendicular L29 L44
  constraint perpendicular L37 L45
  constraint perpendicular L28 L46
  constraint perpendicular L28 L47
  constraint horizontal L50
  constraint midpoint L12 L51.start
  constraint midpoint L10 L51.end
  constraint symmetric L28.start L51 L54.end
  constraint symmetric L28.end L51 L55.end
  constraint symmetric L29.end L51 L56.end
  constraint symmetric L30.end L51 L57.end
  constraint symmetric L31.end L51 L58.end
  constraint symmetric L34.end L51 L52.start
  constraint symmetric L35.end L51 L52.end
  constraint symmetric L36.end L51 L53.end
  constraint symmetric L40.end L51 L63.start
  constraint symmetric L46.end L51 L61.start
  constraint symmetric L47.end L51 L59.end
  constraint symmetric L48.end L51 L60.start
  constraint symmetric L49.start L51 L59.start
  constraint symmetric L41.end L51 L62.start
  constraint symmetric L43.end L51 L64.end
  measures "d107" distance of L39.end L40.end
  measures "d108" distance of L29.end L44.end
  measures "d109" distance of L36.end L45.end
extrude "Extrude26" add sketch "Sketch18" against normal blind 3.5 separate body contours L28 L29 L30 L31 L35 L36 L37 L42 | L52 L53 L54 L55 L56 L57 L58 L67 makes body 6 at (-6.7114, -4, -9.1467) makes body 7 at (6.7114, -4, -9.1467)